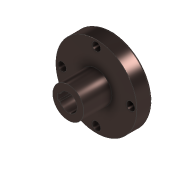
# Autodesk Inventor part: wielhub
Saved by Autodesk Inventor 2020.3 (Build 243373000, 373)
## iProperties
Created: 2020-09-10
Part Number: wielhub
Material: Stainless Steel
Document SubType Name: Modeling
Designer: Svend
Density: 8 g/cm^3
Appearance: Semi-Polished
Author: Svend
Autodesk Inventor part; units mm, degrees
ref_plane "YZ Plane" through (0, 0, 0) normal (1, 0, 0) x (0, 1, 0)
ref_plane "XZ Plane" through (0, 0, 0) normal (0, 1, 0) x (-1, 0, 0)
ref_plane "XY Plane" through (0, 0, 0) normal (0, 0, 1) x (1, 0, 0)
sketch "Sketch1" plane through (0, 0, 0) normal (0, 0, 1) x (1, 0, 0)
  circle A0 centre (0, 0) radius 39
  circle A1 centre (0, 33) radius 4
  circle A2 centre (-33, 0) radius 4
  circle A3 centre (0, -33) radius 4
  circle A4 centre (33, 0) radius 4
  circle A5 centre (0, 0) radius 15
  dimension "d0" = 78
  dimension "d1" = 33
  dimension "d2" = 8
  dimension "d5" = 360
  dimension "d7" = 30
  constraints: 6 centre point, 2 coincident, 1 vertical alignment, 9 other
  measures "d0" diameter of A0
  measures "d1" distance of point (0, 0) A1.centre
  measures "d2" diameter of A1
  measures "d7" diameter of A5
extrude "Extrusion1" add sketch "Sketch1" along normal blind 15
ref_plane "Work Plane1" through (0, 0, 6) normal (0, 0, -1) x (-1, 0, 0)
sketch "Sketch2" plane through (0, 0, 6) normal (0, 0, -1) x (-1, 0, 0)
  circle A0 centre (0, 0) radius 39 projected
  circle A1 centre (0, 0) radius 15 projected
  circle A2 centre (-33, 0) radius 4 projected
  circle A3 centre (0, -33) radius 4 projected
  circle A4 centre (33, 0) radius 4 projected
  circle A5 centre (0, 33) radius 4 projected
  circle A6 centre (0, 0) radius 8.5
  line L0 (7.953, 3) -> (10, 3)
  line L1 (10, 3) -> (10, -3)
  line L2 (10, -3) -> (7.953, -3)
  point P0 (10, 0)
  dimension "d11" = 17
  dimension "d12" = 10
  dimension "d13" = 6
  constraints: 6 end point, 2 perpendicular, 2 point on circle, 1 centre point, 1 coincident, 1 horizontal, 1 horizontal alignment, 1 midpoint
  measures "d11" diameter of A6
  measures "d12" distance from line of point (0, 0) L1
  measures "d13" distance between parallel lines of L0 L2
extrude "Extrusion2" add sketch "Sketch2" against normal blind 36 contours A1
sketch "Sketch3" plane through (0, 0, 0) normal (0, 0, -1) x (-1, 0, 0)
  circle A0 centre (33, 0) radius 4 projected
  circle A1 centre (0, -33) radius 4 projected
  circle A2 centre (-33, 0) radius 4 projected
  circle A3 centre (0, 33) radius 4 projected
  circle A4 centre (0, -33) radius 5.5
  circle A5 centre (-33, 0) radius 5.5
  circle A6 centre (0, 33) radius 5.5
  circle A7 centre (33, 0) radius 5.5
  point P0 (0, 0)
  dimension "d16" = 11
  constraints: 4 centre point, 4 coincident, 3 equal radius
  measures "d16" diameter of A4
extrude "Extrusion3" cut sketch "Sketch3" against normal blind 8 contours A0 | A1 | A2 | A3 | A4 | A5 | A6 | A7
fillet "Fillet1" radius 2 1 edges at (-39, 0, 0)
fillet "Fillet2" radius 0.2 42 edges at (-27.5, 0, 8) (-38.0423, 2.1966, 0.3334) (-38.0423, -2.1966, 0.3334) (-27.5, 0, 0) (0, -38.5, 0.6771) (-5.1089, -35.0369, 0) (2.0369, -27.8911, 0) (-4, -33, 8) (5.5, -33, 8) (-4, -33, 15) (-4, 33, 15) (-37, 0, 15) (-37, 0, 8) (-8.9765, -3, 6) (8.5, 0, 6) (15, 0, 42) (8.5, 0, 42) (-7.953, -3, 24) (-10, -3, 24) (-10, 3, 24) (-7.953, 3, 24) (-8.9765, 3, 6) (38.5, 0, 8) (29, 0, 8) (5.5, 33, 8) (0, 38.5, 0.6771) (-5.1089, 35.0369, 0) (2.0369, 27.8911, 0) (38.0423, 2.1966, 0.3334) (38.0423, -2.1966, 0.3334) (30.8277, 5.0528, 0) (30.8277, -5.0528, 0) (-15, 0, 0) (15, 0, 15) (-15, 0, 6) (-39, 0, 15) (29, 0, 15) (-4, 33, 8) (-10, 0, 6) (-8.9765, 3, 42) (-8.9765, -3, 42) (-10, 0, 42)
body "Solid1"
